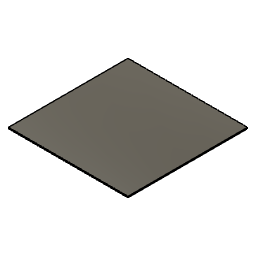
Main model (Autodesk Fusion 360 archive; units mm, degrees)
design "cap"
Autodesk Fusion 360 part; units mm, degrees
sketch "Sketch1" plane through (0, 0, 0) normal (0, 0, 1) x (1, 0, 0)
  line L0 (-75, 80) -> (-75, -80)
  line L1 (-75, -80) -> (75, -80)
  line L2 (75, -80) -> (75, 80)
  line L3 (75, 80) -> (-75, -80) construction
  line L4 (-75, 80) -> (75, -80) construction
  dimension "d1" = 150
  dimension "d2" = 160
  constraint parallel L0 L2
  constraint coincident L3 origin
  constraint coincident L4 origin
  measures "d1" distance of L0.end L1.end
  measures "d2" distance of L0.start L0.end
sketch "Sketch2" plane through (0, 0, 0) normal (0, 0, 1) x (1, 0, 0)
  line L0 (75, -75) -> (-75, -75)
  line L1 (-75, -75) -> (-75, 75)
  line L2 (-75, 75) -> (75, 75)
  line L3 (75, 75) -> (75, -75)
  line L4 (75, -75) -> (-75, 75) construction
  line L5 (-75, -75) -> (75, 75) construction
  dimension "d5" = 150
  dimension "d6" = 150
  constraint horizontal L0
  constraint perpendicular L0 L1
  constraint parallel L0 L2
  constraint parallel L1 L3
  constraint coincident L4 origin
  constraint coincident L5 origin
  measures "d5" distance of L1.end L2.end
  measures "d6" distance of L0.end L1.end
extrude "Extrude2" add sketch "Sketch2" along normal blind 1.5

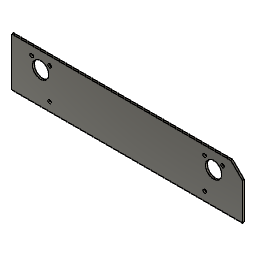
design "motor mount"
Autodesk Fusion 360 part; units mm, degrees
sketch "Sketch15" plane through (0, 0, 0) normal (0, 1, 0) x (1, 0, 0)
  line L0 (100, 21) -> (-100, 21)
  line L1 (-100, 21) -> (-100, -21)
  line L2 (-100, -21) -> (100, -21)
  line L3 (100, -21) -> (100, 21)
  line L4 (100, 21) -> (-100, -21) construction
  line L5 (-100, 21) -> (100, -21) construction
  dimension "d41" = 200
  dimension "d42" = 42
  constraint horizontal L0
  constraint perpendicular L0 L1
  constraint parallel L0 L2
  constraint parallel L1 L3
  constraint coincident L4 origin
  constraint coincident L5 origin
  measures "d41" distance of L1.end L2.end
  measures "d42" distance of L0.end L1.end
extrude "Extrude7" add sketch "Sketch15" along normal blind 1.5
hole "Hole5" at (67.2428, 0, 13.4085) direction (0, 1, 0) diameter 3 depth 7 tip angle 118
hole "Hole6" at (75.0009, 0, 6.5047) direction (0, 1, 0) diameter 14 depth 15 tip angle 118
hole "Hole7" at (82.7411, 0, 13.4378) direction (0, 1, 0) diameter 3 depth 5 tip angle 118
hole "Hole8" at (67.2952, 0, -13.4263) direction (0, 1, 0) diameter 3 depth 6 tip angle 118
sketch "Sketch16" plane through (0, 0, 0) normal (1, 0, 0) x (0, 1, 0)
  line L0 (-56.4532, 39.0008) -> (75, 39.0008)
  line L1 (75, 39.0008) -> (75, -35)
  line L2 (75, -35) -> (-56.4532, -35)
  line L3 (-56.4532, -35) -> (-56.4532, 39.0008)
  constraint horizontal L0
  constraint vertical L1
  constraint horizontal L2
  constraint vertical L3
ref_plane "WorkPlane2" through (0, 9.2734, 2.0004) normal (1, 0, 0) x (0, 1, 0)
mirror "Mirror1" about plane through (0, 9.2734, 2.0004) normal (1, 0, 0) of "Hole5", "Hole6", "Hole7", "Hole8"
chamfer "Chamfer1" distance 10 angle 45 1 edges at (100, 0.75, 21)

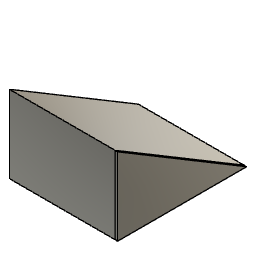
design "clamp"
Autodesk Fusion 360 part; units mm, degrees
sketch "Sketch8" plane through (0, 0, 0) normal (1, 0, 0) x (0, 1, 0)
  line L0 (0, 0) -> (0, -30)
  line L1 (0, -30) -> (50, -30)
  line L2 (50, -30) -> (0, 0)
  line L3 (0, -30, 50) -> (50, -30, 50)
  line L4 (50, -30, 50) -> (0, 0, 50)
  line L5 (0, 0, 50) -> (0, -30, 50)
  dimension "d23" = 30
  dimension "d24" = 50
  dimension "d28" = 30
  dimension "d29" = 50
  constraint coincident L0.start L2.end
  constraint vertical L0
  constraint perpendicular L0 L1
  measures "d23" distance of L0.start L0.end
  measures "d24" distance of L0.end L1.end
  measures "d28" distance of L0.end L0.start
  measures "d29" distance of L1.end L0.end
extrude "Extrude6" add sketch "Sketch8" along normal blind 40 thin wall 1 inside makes body 1
sketch "Sketch9" plane through (0, 0, 0) normal (1, 0, 0) x (0, 1, 0)
  line L0 (0, 0) -> (0, -30)
  line L1 (0, -30) -> (50, -30)
  line L2 (50, -30) -> (0, 0)
  constraint coincident L0.start L2.end
  constraint vertical L0
  constraint perpendicular L0 L1
extrude "Extrude7" add sketch "Sketch9" against normal blind 1 separate body makes body 2
move_body "Move1" bodies 2 to x (1, 0, 0) y (0, 1, 0) z (0, 0, 1) at (41, 0, 0)
extrude "Extrude8" add sketch "Sketch8" against normal blind 1 bodies 1
move_body "Move2" bodies 2 1 to x (1, 0, 0) y (0, 1, 0) z (0, 0, 1) at (-5, -10, 0)
